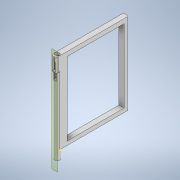
# Autodesk Inventor part: door
Saved by Autodesk Inventor 2022.5 (Build 265521000, 521)
## iProperties
Created: 2025-01-06
Part Number: door
Material: 常规
Document SubType Name: Modeling
Designer: Administrator
Density: 1 g/cm^3
Appearance: 默认
Mass: 49.4459 g
Surface Area: 190.975 cm^2
Volume: 49.4459 cm^3
Author: Administrator
Autodesk Inventor part; units mm, degrees
ref_plane "YZ Plane" through (0, 0, 0) normal (1, 0, 0) x (0, 1, 0)
ref_plane "XZ Plane" through (0, 0, 0) normal (0, 1, 0) x (-1, 0, 0)
ref_plane "XY Plane" through (0, 0, 0) normal (0, 0, 1) x (1, 0, 0)
sketch "草图1" plane through (0, 0, 0) normal (0, 1, 0) x (-1, 0, 0)
  line L0 (0, 0) -> (6, 0)
  line L1 (6, 0) -> (6, -80)
  line L2 (6, -80) -> (0, -80)
  line L3 (0, -80) -> (0, 0)
  dimension "d0" = 6
  dimension "d1" = 80
  constraints: 8 end point, 2 parallel, 1 horizontal, 1 perpendicular
  measures "d0" distance of L1.end L2.end
  measures "d1" distance of L0.end L1.end
extrude "拉伸1" add sketch "草图1" along normal blind 95
sketch "草图7" plane through (0, 95, 0) normal (0, 1, 0) x (1, 0, 0)
  line L0 (-6, 0) -> (0, 0) projected
  circle A0 centre (-3, 0) radius 3
  constraints: 1 horizontal alignment, 1 midpoint, 2 other
extrude "拉伸6" add sketch "草图7" against normal up to surface (95 mm away)
sketch "草图8" plane through (0, 0, 0) normal (0, -1, 0) x (1, 0, 0)
  line L0 (-6, -80) -> (-6, 0) projected
  line L1 (0, -80) -> (-6, -80) projected
  line L2 (0, 0) -> (0, -80) projected
  arc A0 (0, 0) -> (-6, 0) centre (-3, 0) ccw projected
  line L3 (0, 0) -> (0, -80) projected
  circle A1 centre (-3, 0) radius 3
  point P0 (-6, 0)
  constraints: 1 coincident, 3 other
extrude "拉伸7" add sketch "草图8" along normal blind 10 contours A0 A1
ref_plane "工作平面1" through (-3, 95, 3) normal (0, 0, -1) x (-1, 0, 0)
sketch "草图11" plane through (0, 95, 0) normal (0, 1, 0) x (1, 0, 0)
  line L0 (0, 0) -> (0, 80) projected
  line L1 (0, 80) -> (-6, 80) projected
  line L2 (-6, 80) -> (-6, 0) projected
  arc A0 (-6, 0) -> (0, 0) centre (-3, 0) ccw projected
  circle A1 centre (-3, 0) radius 2.5
  line L3 (-1.5, -2) -> (-4.5, -2)
  dimension "d27" = 5
  dimension "d28" = 4.5
  constraints: 2 end point, 2 point on circle, 1 centre point, 1 coincident, 1 horizontal
  measures "d27" diameter of A1
extrude "拉伸9" cut sketch "草图11" against normal blind 25 contours A1 L3 picked at (-2.3724, -0.7851)
sketch "草图12" plane through (-3, 95, 3) normal (0, 0, -1) x (-1, 0, 0)
  line L0 (-3, -105) -> (3, -105) projected
  line L1 (-3, -95) -> (-3, 0) projected
  line L2 (3, 0) -> (-3, 0) projected
  line L3 (3, -95) -> (3, 0) projected
  line L4 (-3, -95) -> (3, -95) projected
  line L5 (-3, -95) -> (-3, 0) projected
  line L6 (3, 0) -> (-3, 0) projected
  line L7 (-3, -16.1112) -> (3, -16.1112)
  line L8 (3, -16.1112) -> (3, 0)
  line L9 (3, 0) -> (-3, 0)
  line L10 (-3, 0) -> (-3, -16.1112)
  constraints: 8 end point, 2 parallel, 1 horizontal, 1 perpendicular, 1 point on line
extrude "拉伸10" add sketch "草图12" along normal up to surface contours L1 L2 L3 L7 round surface about axis through (-3, 95, 0) along (0, -1, 0) radius 3 far side no
sketch "草图13" plane through (-3, 95, 3) normal (0, 0, 1) x (1, 0, 0)
  line L0 (3, -16.1112) -> (0, -16.1112) projected
  line L1 (3, 0) -> (3, -16.1112) projected
  line L2 (-3, 0) -> (3, 0) projected
  line L3 (-3, -16.1112) -> (-3, 0) projected
  line L4 (0, -16.1112) -> (-3, -16.1112) projected
  point P0 (3, -95)
extrude "拉伸11" add sketch "草图13" along normal blind 1
sketch "草图14" plane through (-3, 95, 4) normal (0, 0, 1) x (1, 0, 0)
  line L0 (3, 0) -> (-3, 0) projected
  line L1 (-3, 0) -> (-3, -16.1112) projected
  line L2 (-3, -16.1112) -> (3, -16.1112) projected
  line L3 (3, -16.1112) -> (3, 0) projected
  point P0 (3, -95)
  point P1 (0, -3.0228)
hole "孔1" at (-3, 91.9772, 4) direction (0, 0, -1) diameter 2.459 depth 6.3 thread size "M3x0.5" designation "M3" class "6H" standard "GB Metric profile"
fillet "圆角1" radius 2 2 edges at (-6, 86.9444, 4) (0, 86.9444, 4)
sketch "草图15" plane through (0, 0, -80) normal (1, 0, 0) x (0, 0, -1)
  line L0 (-5.5, 5) -> (-71.683, 5)
  line L1 (-71.683, 5) -> (-71.683, 90)
  line L2 (-71.683, 90) -> (-5.5, 90)
  line L3 (-5.5, 90) -> (-5.5, 5)
  line L4 (0, 0) -> (0, 95) projected
  line L5 (-80, 0) -> (0, 0) projected
  line L6 (-82, 95) -> (0, 95) projected
  dimension "d43" = 5.5
  dimension "d44" = 5
  dimension "d45" = 5
  constraints: 8 end point, 2 parallel, 1 horizontal, 1 perpendicular
  measures "d43" distance between parallel lines of L4 L3
  measures "d44" distance between parallel lines of L5 L0
  measures "d45" distance between parallel lines of L6 L2
extrude "拉伸12" cut sketch "草图15" against normal blind 28.5
fillet "圆角2" radius 2 2 edges at (-6, 47.5, -80) (0, 47.5, -80)
sketch "草图16" plane through (-3, 95, 4) normal (0, 0, 1) x (1, 0, 0)
  line L0 (-1, -2.3075) -> (-1, 0) projected
  line L1 (-1, 0) -> (-3, 0) projected
  line L2 (-3, 0) -> (-3, -16.1112) projected
  line L3 (-3, -16.1112) -> (-1, -16.1112) projected
  line L4 (-1, -16.1112) -> (-1, -3.7382) projected
  line L5 (1, -3.7382) -> (1, -16.1112) projected
  arc A0 (-1, -3.7382) -> (1, -3.7382) centre (0, -3.0228) ccw projected
  line L6 (-1, -16.1112) -> (-1, -3.7382) projected
  line L7 (-1, -16.1112) -> (1, -16.1112) projected
  line L8 (2.5, 0) -> (2.5, -25) projected
  line L9 (1, -3.7382) -> (1, -16.1112) projected
  line L10 (1, -16.1112) -> (3, -16.1112) projected
  line L11 (3, -16.1112) -> (3, 0) projected
  line L12 (3, 0) -> (1, 0) projected
  line L13 (1, 0) -> (1, -2.3075) projected
  line L14 (-1.5, 0) -> (-1.5, -25) projected
  line L15 (1.5, 0) -> (1.5, -25) projected
  line L16 (-1.5, -5.3722) -> (1.5, -5.3722)
  line L17 (1.5, -5.3722) -> (1.5, -15.0764)
  line L18 (1.5, -15.0764) -> (-1.5, -15.0764)
  line L19 (-1.5, -15.0764) -> (-1.5, -5.3722)
  point P0 (3, -95)
  point P1 (-1.5, -15.0764)
  constraints: 8 end point, 2 parallel, 2 point on line, 2 vertical alignment, 1 horizontal, 1 perpendicular
extrude "拉伸13" cut sketch "草图16" against normal blind 4.5 contours L16 L4 L18 L14 | L16 L5 L18 L4 | L16 L15 L18 L5
sketch "草图17" plane through (-1.5, 70, 2) normal (0, 0, -1) x (-1, 0, 0)
  line L0 (-1.5, 8.8888) -> (4.5, 8.8888) projected
  line L1 (4.5, -70) -> (4.5, 8.8888) projected
  line L2 (-1.5, -70) -> (4.5, -70) projected
  line L3 (-1.5, -70) -> (-1.5, 8.8888) projected
  line L4 (-1.5, -80) -> (4.5, -80) projected
  line L5 (3, 9.9236) -> (3, 0) projected
  line L6 (0, 0) -> (3, 0) projected
  line L7 (3, 8.8888) -> (0, 8.8888)
  line L8 (0, 8.8888) -> (0, 0)
  line L9 (0, 0) -> (3, 0)
  line L10 (3, 0) -> (3, 8.8888)
  constraints: 8 end point, 2 parallel, 2 point on line, 1 horizontal, 1 perpendicular
extrude "拉伸14" cut sketch "草图17" against normal blind 2.25 contours L0 L5 L6 L8
sketch "草图18" plane through (0, 0, 0) normal (1, 0, 0) x (0, 0, -1)
  point P0 (0, 0)
chamfer "倒角2" distance 0.5 angle 45 5 edges at (0, 0, -39) (-0.5858, 0, -79.4142) (-3, 0, -80) (-5.4142, 0, -79.4142) (-6, 0, -39)
